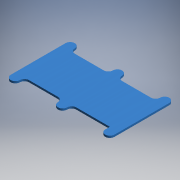
# Autodesk Inventor part: Body_bottom
Saved by Autodesk Inventor 2017 (Build 210142000, 142)
## iProperties
Part Number: Body_bottom
Material: Generic
Document SubType Name: Modeling
Designer: alex-
Appearance: Cyan
Author: alex-
Autodesk Inventor part; units mm, degrees
ref_plane "YZ Plane" through (0, 0, 0) normal (1, 0, 0) x (0, 1, 0)
ref_plane "XZ Plane" through (0, 0, 0) normal (0, 1, 0) x (-1, 0, 0)
ref_plane "XY Plane" through (0, 0, 0) normal (0, 0, 1) x (1, 0, 0)
sketch "Sketch1" plane through (0, 0, 0) normal (0, 1, 0) x (-1, 0, 0)
  line L0 (136, 84) -> (112, 84)
  line L1 (136, -84) -> (112, -84)
  line L2 (136, 84) -> (136, -84)
  line L3 (112, 84) -> (112, 60)
  line L4 (112, -60) -> (112, -84)
  line L5 (112, 60) -> (12, 60)
  line L6 (112, -60) -> (12, -60)
  line L7 (12, 60) -> (12, 84)
  line L8 (12, -60) -> (12, -84)
  line L9 (12, 84) -> (-12, 84)
  line L10 (12, -84) -> (-12, -84)
  line L11 (-12, 84) -> (-12, 60)
  line L12 (-12, -60) -> (-12, -84)
  line L13 (-12, 60) -> (-112, 60)
  line L14 (-12, -60) -> (-112, -60)
  line L15 (-112, 60) -> (-112, 84)
  line L16 (-112, -60) -> (-112, -84)
  line L17 (-112, 84) -> (-136, 84)
  line L18 (-112, -84) -> (-136, -84)
  line L19 (-136, 84) -> (-136, -84)
  line L20 (136, 0) -> (-136, 0) construction
  line L21 (0, 84) -> (0, -84) construction
  point P0 (0, 0)
  point P1 (0, 0)
  dimension "d0" = 168
  dimension "d1" = 24
  dimension "d3" = 100
  dimension "d4" = 24
  dimension "d5" = 120
  constraints: 44 end point, 16 equal length, 9 vertical, 8 horizontal, 6 horizontal alignment, 5 midpoint, 1 coincident, 1 parallel, 1 perpendicular
  measures "d0" distance of L0.start L1.start
  measures "d1" distance of L0.start L0.end
  measures "d3" distance of L3.end L5.end
  measures "d4" distance of L0.end L3.end
  measures "d5" distance between parallel lines of L6 L5
extrude "Extrusion1" add sketch "Sketch1" along normal blind 5
fillet "Fillet1" radius 12 19 edges at (-136, 2.5, 84) (-112, 2.5, 84) (-112, 2.5, 60) (112, 2.5, 84) (136, 2.5, 84) (12, 2.5, 84) (-12, 2.5, 84) (12, 2.5, 60) (-12, 2.5, 60) (-136, 2.5, -84) (-112, 2.5, -84) (-12, 2.5, -60) (-12, 2.5, -84) (12, 2.5, -84) (112, 2.5, -60) (112, 2.5, -84) (136, 2.5, -84) (12, 2.5, -60) (-112, 2.5, -60)
equation "\"d1\" = sa_diameter"
equation "\"d3\" = b_leg_space"
equation "\"d4\" = sa_diameter"
equation "\"d5\" = b_core_width"
equation "\"d6\" = b_mat_thickness"
equation "\"d22\" = 0.5 * sa_diameter"
equation "\"sa_diameter\" = 24"
equation "\"b_leg_space\" = 100"
equation "\"b_core_width\" = 120"
equation "\"b_mat_thickness\" = 5"
body "Solid1"
